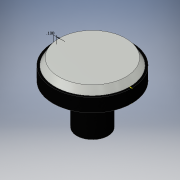
# Autodesk Inventor part: ButtonLarge
Saved by Autodesk Inventor 2016 (Build 200138000, 138)
## iProperties
Created: 2017-01-21
Part Number: ButtonLarge
Material: Generic
Document SubType Name: Modeling
Designer: Owner
Density: 1 g/cm^3
Appearance: Default
Author: Owner
Autodesk Inventor part; units mm, degrees
ref_plane "YZ Plane" through (0, 0, 0) normal (1, 0, 0) x (0, 1, 0)
ref_plane "XZ Plane" through (0, 0, 0) normal (0, 1, 0) x (-1, 0, 0)
ref_plane "XY Plane" through (0, 0, 0) normal (0, 0, 1) x (1, 0, 0)
sketch "Sketch1" plane through (0, 0, 0) normal (0, 1, 0) x (-1, 0, 0)
  line L0 (0, -41.9252) -> (0, 41.9252) projected
  line L1 (-41.9252, 0) -> (41.9252, 0) projected
  circle A0 centre (0, 0) radius 29.9466
  dimension "d0" = 59.8932
  constraints: 1 centre point, 1 coincident
  measures "d0" diameter of A0
extrude "Extrusion1" add sketch "Sketch1" along normal blind 10.16
sketch "Sketch2" plane through (0, 0, 0) normal (0, 0, 1) x (1, 0, 0)
  line L0 (-29.9466, 0) -> (29.9466, 0) projected
  line L1 (29.9466, 10.16) -> (-29.9466, 10.16) projected
  line L2 (-29.9466, 0) -> (0, 0)
  line L3 (0, 0) -> (0, 10.16)
  line L4 (0, 10.16) -> (-29.9466, 10.16)
  line L5 (-29.9466, 10.16) -> (-29.9466, 0)
  line L6 (-29.9466, 0) -> (-27.4066, 10.16)
  line L7 (-29.9466, 10.16) -> (-27.4066, 10.16)
  dimension "d4" = 2.54
  constraints: 12 end point, 2 parallel, 1 collinear, 1 horizontal, 1 midpoint, 1 perpendicular, 1 point on line
  measures "d4" distance of L4.end L6.end
sketch "Sketch3" plane through (0, 10.16, 0) normal (0, 1, 0) x (1, 0, 0)
  circle A0 centre (0, 0) radius 25.4
  dimension "d8" = 50.8
  constraints: 1 centre point, 1 coincident
  measures "d8" diameter of A0
extrude "Extrusion2" add sketch "Sketch3" along normal blind 5.08
draft "FaceDraft1" angle -30 pull direction (0, -1, 0) faces at (25.3176, 13.5467, 2.0439) fixed edges at (-25.4, 15.24, 0)
sketch "Sketch4" plane through (0, 0, 0) normal (0, -1, 0) x (1, 0, 0)
  circle A0 centre (0, 0) radius 11.811
  dimension "d9" = 23.622
  constraints: 1 centre point, 1 coincident
  measures "d9" diameter of A0
extrude "Extrusion3" add sketch "Sketch4" along normal blind 30.48
body "Solid1"
